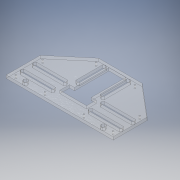
# Autodesk Inventor part: phone_holder_back_back
Saved by Autodesk Inventor 2019 (Build 230136000, 136)
## iProperties
Created: 2019-02-17
Part Number: phone_holder_back_back
Material: Acrylic, Clear
Document SubType Name: Modeling
Designer: suchanek
Density: 1.19 g/cm^3
Appearance: Transparent - Clear
Author: suchanek
Autodesk Inventor part; units mm, degrees
ref_plane "YZ Plane" through (0, 0, 0) normal (1, 0, 0) x (0, 1, 0)
ref_plane "XZ Plane" through (0, 0, 0) normal (0, 1, 0) x (-1, 0, 0)
ref_plane "XY Plane" through (0, 0, 0) normal (0, 0, 1) x (1, 0, 0)
sketch "Sketch2" plane through (0, 0, 0) normal (0, 1, 0) x (-1, 0, 0)
  line L0 (110, 62.5) -> (-110, 62.5)
  line L1 (-110, 62.5) -> (-110, -62.5)
  line L2 (-110, -62.5) -> (110, -62.5)
  line L3 (110, -62.5) -> (110, 62.5)
  line L4 (110, 62.5) -> (-110, -62.5) construction
  line L5 (-110, 62.5) -> (110, -62.5) construction
  line L6 (11.5, -50.5) -> (17.5, -50.5)
  line L7 (17.5, -50.5) -> (17.5, -38.5)
  line L8 (17.5, -38.5) -> (11.5, -38.5)
  line L9 (11.5, -38.5) -> (11.5, -50.5)
  line L10 (11.5, -26.5) -> (17.5, -26.5)
  line L11 (17.5, -26.5) -> (17.5, -14.5)
  line L12 (17.5, -14.5) -> (11.5, -14.5)
  line L13 (11.5, -14.5) -> (11.5, -26.5)
  line L14 (11.5, -2.5) -> (17.5, -2.5)
  line L15 (17.5, -2.5) -> (17.5, 9.5)
  line L16 (17.5, 9.5) -> (11.5, 9.5)
  line L17 (11.5, 9.5) -> (11.5, -2.5)
  line L18 (-17.5, -50.5) -> (-11.5, -50.5)
  line L19 (-11.5, -50.5) -> (-11.5, -38.5)
  line L20 (-11.5, -38.5) -> (-17.5, -38.5)
  line L21 (-17.5, -38.5) -> (-17.5, -50.5)
  line L22 (-17.5, -26.5) -> (-11.5, -26.5)
  line L23 (-11.5, -26.5) -> (-11.5, -14.5)
  line L24 (-11.5, -14.5) -> (-17.5, -14.5)
  line L25 (-17.5, -14.5) -> (-17.5, -26.5)
  line L26 (-17.5, -2.5) -> (-11.5, -2.5)
  line L27 (-11.5, -2.5) -> (-11.5, 9.5)
  line L28 (-11.5, 9.5) -> (-17.5, 9.5)
  line L29 (-17.5, 9.5) -> (-17.5, -2.5)
  line L30 (0, 0) -> (0, -18.9718)
  line L31 (25, -2.5) -> (25, -52.5) construction
  line L32 (21, -2.5) -> (21, -52.5)
  line L33 (29, -52.5) -> (29, -2.5)
  arc A0 (29, -2.5) -> (21, -2.5) centre (25, -2.5) ccw
  arc A1 (21, -52.5) -> (29, -52.5) centre (25, -52.5) ccw
  line L34 (100, 12.5) -> (40, 12.5) construction
  line L35 (100, 16.5) -> (40, 16.5)
  line L36 (40, 8.5) -> (100, 8.5)
  arc A2 (100, 8.5) -> (100, 16.5) centre (100, 12.5) ccw
  arc A3 (40, 16.5) -> (40, 8.5) centre (40, 12.5) ccw
  line L37 (100, 37.5) -> (40, 37.5) construction
  line L38 (100, 41.5) -> (40, 41.5)
  line L39 (40, 33.5) -> (100, 33.5)
  arc A4 (100, 33.5) -> (100, 41.5) centre (100, 37.5) ccw
  arc A5 (40, 41.5) -> (40, 33.5) centre (40, 37.5) ccw
  line L40 (-25, -2.5) -> (-25, -52.5) construction
  line L41 (-21, -2.5) -> (-21, -52.5)
  line L42 (-29, -52.5) -> (-29, -2.5)
  arc A6 (-21, -2.5) -> (-29, -2.5) centre (-25, -2.5) ccw
  arc A7 (-29, -52.5) -> (-21, -52.5) centre (-25, -52.5) ccw
  line L43 (-100, 12.5) -> (-40, 12.5) construction
  line L44 (-100, 16.5) -> (-40, 16.5)
  line L45 (-40, 8.5) -> (-100, 8.5)
  arc A8 (-100, 16.5) -> (-100, 8.5) centre (-100, 12.5) ccw
  arc A9 (-40, 8.5) -> (-40, 16.5) centre (-40, 12.5) ccw
  line L46 (-100, 37.5) -> (-40, 37.5) construction
  line L47 (-100, 41.5) -> (-40, 41.5)
  line L48 (-40, 33.5) -> (-100, 33.5)
  arc A10 (-100, 41.5) -> (-100, 33.5) centre (-100, 37.5) ccw
  arc A11 (-40, 33.5) -> (-40, 41.5) centre (-40, 37.5) ccw
  circle A12 centre (80, 52.5) radius 4
  circle A13 centre (-80, 52.5) radius 4
  line L49 (110, -7.5) -> (45, -62.5)
  line L50 (-45, -62.5) -> (-110, -7.5)
  line L51 (29, -4.8094) -> (25, -7.1188)
  line L52 (25, -7.1188) -> (21, -4.8094)
  line L53 (21, -4.8094) -> (21, -0.1906)
  line L54 (21, -0.1906) -> (25, 2.1188)
  line L55 (25, 2.1188) -> (29, -0.1906)
  line L56 (29, -0.1906) -> (29, -4.8094)
  line L57 (29, -54.8094) -> (25, -57.1188)
  line L58 (25, -57.1188) -> (21, -54.8094)
  line L59 (21, -54.8094) -> (21, -50.1906)
  line L60 (21, -50.1906) -> (25, -47.8812)
  line L61 (25, -47.8812) -> (29, -50.1906)
  line L62 (29, -50.1906) -> (29, -54.8094)
  line L63 (-21, -54.8094) -> (-25, -57.1188)
  line L64 (-25, -57.1188) -> (-29, -54.8094)
  line L65 (-29, -54.8094) -> (-29, -50.1906)
  line L66 (-29, -50.1906) -> (-25, -47.8812)
  line L67 (-25, -47.8812) -> (-21, -50.1906)
  line L68 (-21, -50.1906) -> (-21, -54.8094)
  line L69 (-21, -4.8094) -> (-25, -7.1188)
  line L70 (-25, -7.1188) -> (-29, -4.8094)
  line L71 (-29, -4.8094) -> (-29, -0.1906)
  line L72 (-29, -0.1906) -> (-25, 2.1188)
  line L73 (-25, 2.1188) -> (-21, -0.1906)
  line L74 (-21, -0.1906) -> (-21, -4.8094)
  line L75 (-42.3094, 8.5) -> (-44.6188, 12.5)
  line L76 (-44.6188, 12.5) -> (-42.3094, 16.5)
  line L77 (-42.3094, 16.5) -> (-37.6906, 16.5)
  line L78 (-37.6906, 16.5) -> (-35.3812, 12.5)
  line L79 (-35.3812, 12.5) -> (-37.6906, 8.5)
  line L80 (-37.6906, 8.5) -> (-42.3094, 8.5)
  line L81 (-42.3094, 33.5) -> (-44.6188, 37.5)
  line L82 (-44.6188, 37.5) -> (-42.3094, 41.5)
  line L83 (-42.3094, 41.5) -> (-37.6906, 41.5)
  line L84 (-37.6906, 41.5) -> (-35.3812, 37.5)
  line L85 (-35.3812, 37.5) -> (-37.6906, 33.5)
  line L86 (-37.6906, 33.5) -> (-42.3094, 33.5)
  line L87 (-102.3094, 33.5) -> (-104.6188, 37.5)
  line L88 (-104.6188, 37.5) -> (-102.3094, 41.5)
  line L89 (-102.3094, 41.5) -> (-97.6906, 41.5)
  line L90 (-97.6906, 41.5) -> (-95.3812, 37.5)
  line L91 (-95.3812, 37.5) -> (-97.6906, 33.5)
  line L92 (-97.6906, 33.5) -> (-102.3094, 33.5)
  line L93 (-102.3094, 8.5) -> (-104.6188, 12.5)
  line L94 (-104.6188, 12.5) -> (-102.3094, 16.5)
  line L95 (-102.3094, 16.5) -> (-97.6906, 16.5)
  line L96 (-97.6906, 16.5) -> (-95.3812, 12.5)
  line L97 (-95.3812, 12.5) -> (-97.6906, 8.5)
  line L98 (-97.6906, 8.5) -> (-102.3094, 8.5)
  line L99 (-82.3094, 48.5) -> (-84.6188, 52.5)
  line L100 (-84.6188, 52.5) -> (-82.3094, 56.5)
  line L101 (-82.3094, 56.5) -> (-77.6906, 56.5)
  line L102 (-77.6906, 56.5) -> (-75.3812, 52.5)
  line L103 (-75.3812, 52.5) -> (-77.6906, 48.5)
  line L104 (-77.6906, 48.5) -> (-82.3094, 48.5)
  line L105 (77.6906, 48.5) -> (75.3812, 52.5)
  line L106 (75.3812, 52.5) -> (77.6906, 56.5)
  line L107 (77.6906, 56.5) -> (82.3094, 56.5)
  line L108 (82.3094, 56.5) -> (84.6188, 52.5)
  line L109 (84.6188, 52.5) -> (82.3094, 48.5)
  line L110 (82.3094, 48.5) -> (77.6906, 48.5)
  line L111 (97.6906, 33.5) -> (95.3812, 37.5)
  line L112 (95.3812, 37.5) -> (97.6906, 41.5)
  line L113 (97.6906, 41.5) -> (102.3094, 41.5)
  line L114 (102.3094, 41.5) -> (104.6188, 37.5)
  line L115 (104.6188, 37.5) -> (102.3094, 33.5)
  line L116 (102.3094, 33.5) -> (97.6906, 33.5)
  line L117 (102.3094, 16.5) -> (104.6188, 12.5)
  line L118 (104.6188, 12.5) -> (102.3094, 8.5)
  line L119 (102.3094, 8.5) -> (97.6906, 8.5)
  line L120 (97.6906, 8.5) -> (95.3812, 12.5)
  line L121 (95.3812, 12.5) -> (97.6906, 16.5)
  line L122 (97.6906, 16.5) -> (102.3094, 16.5)
  line L123 (42.3094, 16.5) -> (44.6188, 12.5)
  line L124 (44.6188, 12.5) -> (42.3094, 8.5)
  line L125 (42.3094, 8.5) -> (37.6906, 8.5)
  line L126 (37.6906, 8.5) -> (35.3812, 12.5)
  line L127 (35.3812, 12.5) -> (37.6906, 16.5)
  line L128 (37.6906, 16.5) -> (42.3094, 16.5)
  line L129 (37.6906, 33.5) -> (35.3812, 37.5)
  line L130 (35.3812, 37.5) -> (37.6906, 41.5)
  line L131 (37.6906, 41.5) -> (42.3094, 41.5)
  line L132 (42.3094, 41.5) -> (44.6188, 37.5)
  line L133 (44.6188, 37.5) -> (42.3094, 33.5)
  line L134 (42.3094, 33.5) -> (37.6906, 33.5)
  line L135 (17.5, 9.5) -> (17.5, 14.5)
  line L136 (17.5, -56.5) -> (-17.5, -56.5)
  line L137 (-17.5, -56.5) -> (-17.5, 14.5)
  line L138 (27.5, 34.5) -> (-27.5, 34.5)
  line L139 (-27.5, 34.5) -> (-27.5, 14.5)
  line L140 (-27.5, 14.5) -> (-17.5, 14.5)
  line L141 (27.5, 14.5) -> (27.5, 34.5)
  circle A14 centre (100, 52.5) radius 1.5
  circle A15 centre (40, 52.5) radius 1.5
  circle A16 centre (100, -2.5) radius 1.5
  circle A17 centre (40, -52.5) radius 1.5
  circle A18 centre (-100, 52.5) radius 1.5
  circle A19 centre (-40, 52.5) radius 1.5
  circle A20 centre (-100, -2.5) radius 1.5
  circle A21 centre (-40, -52.5) radius 1.5
  line L142 (17.5, 14.5) -> (17.5, -56.5)
  line L143 (17.5, 14.5) -> (27.5, 14.5)
  line L144 (-17.5, 14.5) -> (17.5, 14.5)
  line L145 (-17.5, 14.5) -> (-17.5, 9.5)
  line L146 (-17.5, -56.5) -> (17.5, -56.5)
  line L147 (17.5, -56.5) -> (17.5, 14.5)
  line L148 (17.5, 14.5) -> (-17.5, 14.5)
  line L149 (-17.5, 14.5) -> (-17.5, -56.5)
  point P0 (25, -27.5)
  point P1 (70, 12.5)
  point P2 (70, 37.5)
  point P3 (-25, -27.5)
  point P4 (-70, 12.5)
  point P5 (-70, 37.5)
  point P6 (-80, 48.5)
  point P7 (80, 48.5)
  dimension "d52" = 220
  dimension "d53" = 125
  dimension "d54" = 12
  dimension "d55" = 6
  dimension "d58" = 24
  dimension "d61" = 29
  dimension "d65" = 12
  dimension "d66" = 8
  dimension "d68" = 100
  dimension "d69" = 115
  dimension "d70" = 40
  dimension "d71" = 65
  dimension "d72" = 15
  dimension "d73" = 25
  dimension "d75" = 15
  dimension "d79" = 30
  dimension "d80" = 10
  dimension "d81" = 20
  dimension "d82" = 20
  dimension "d83" = 6
  dimension "d85" = 20
  dimension "d86" = 10
  dimension "d87" = 10
  dimension "d88" = 3
  dimension "d89" = 5
  constraints: 312 end point, 27 symmetric about line, 24 point on circle, 20 centre point, 19 midpoint, 15 parallel, 14 coincident, 12 tangent, 8 point on line, 8 vertical alignment, 6 horizontal, 6 vertical, 5 equal radius, 5 horizontal alignment, 5 perpendicular, 1 collinear, 238 other
  measures "d52" distance of L2.end L1.end
  measures "d53" distance of L1.end L0.end
  measures "d54" distance of L8.end L6.start
  measures "d55" distance of L6.start L6.end
  measures "d58" distance of L6.start L10.start
  measures "d61" distance of L6.start L18.start
  measures "d65" distance between parallel lines of L2 L6
  measures "d66" diameter of A1
  measures "d68" distance from line of L30 L34.start
  measures "d69" distance from line of L0 L31.end
  measures "d70" distance from line of L30 L34.end
  measures "d71" distance from line of L0 L31.start
  measures "d72" horizontal distance of L31.start L34.end
  measures "d73" distance from line of L0 L37.end
  measures "d75" horizontal distance of L31.start L34.end
  measures "d79" distance from line of L3 point (80, 52.5)
  measures "d80" distance from line of L0 point (80, 52.5)
  measures "d81" distance from line of L49.end L31
  measures "d82" distance from line of L49.start L34
  measures "d83" distance between parallel lines of L136 L18
  measures "d85" distance of L141.start L138.start
  measures "d86" distance between parallel lines of L15 L141
  measures "d87" distance between parallel lines of L29 L139
  measures "d88" diameter of A14
  measures "d89" distance between parallel lines of L16 L144
extrude "Extrusion2" add sketch "Sketch2" along normal blind 6 contours L3 L49 L2 L50 L1 L0
body "Solid2"
